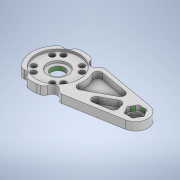
# Autodesk Inventor part: Ankle_side_pitch_frame
Saved by Autodesk Inventor 2020 (Build 240168000, 168)
## iProperties
Part Number: Ankle_side_pitch_frame
Material: アルミニウム 2014-T4
Document SubType Name: Modeling
Designer: Masato Kubotera
Density: 2.8 g/cm^3
Appearance: 滑らか - 淡い灰色
Description: A2017 T4
Mass: 7.07443 g
Surface Area: 29.7848 cm^2
Volume: 2.52658 cm^3
Author: Masato Kubotera
Autodesk Inventor part; units mm, degrees
ref_plane "YZ Plane" through (0, 0, 0) normal (1, 0, 0) x (0, 1, 0)
ref_plane "XZ Plane" through (0, 0, 0) normal (0, 1, 0) x (-1, 0, 0)
ref_plane "XY Plane" through (0, 0, 0) normal (0, 0, 1) x (1, 0, 0)
sketch "スケッチ1" plane through (0, 0, 0) normal (0, 0, 1) x (1, 0, 0)
  circle A0 centre (0, 0) radius 10.5 construction
  circle A1 centre (0, 0) radius 5 construction
  circle A2 centre (0, 0) radius 5.01
  circle A3 centre (0, 0) radius 10.51
  arc A4 (2.1531, 12.3132) -> (2.1531, -12.3132) centre (0, 0) ccw
  circle A5 centre (37.7359, 0) radius 2.75
  arc A6 (38.7694, -5.9103) -> (38.7694, 5.9103) centre (37.7359, 0) ccw
  line L0 (2.1531, 12.3132) -> (38.7694, 5.9103)
  line L1 (2.1531, -12.3132) -> (38.7694, -5.9103)
  line L2 (13.3804, 8.3196) -> (26.7879, 5.9751)
  line L3 (30.7947, -5.2745) -> (23.5904, -6.5342)
  arc A7 (2.1531, -12.3132) -> (-4.7001, 11.5827) centre (0, 0) ccw construction
  arc A8 (38.7694, 5.9103) -> (32.2717, -2.4783) centre (37.7359, 0) ccw construction
  line L4 (34.0196, 4.7105) -> (8.4896, -9.1748) construction
  line L5 (27.399, 2.248) -> (15.2168, -4.3777)
  line L6 (28.8431, 0.7568) -> (22.2903, -2.8072)
  line L7 (32.4358, 4.9875) -> (34.0196, 4.7105) construction
  line L8 (11.5743, -8.6354) -> (8.4896, -9.1748) construction
  arc A9 (31.783, -0.7501) -> (32.2717, -2.4783) centre (37.7359, 0) ccw
  arc A10 (12.2941, -2.2592) -> (11.2378, 5.4737) centre (0, 0) ccw
  line L9 (41.7889, 0) -> (41.2639, -0.9093) construction
  line L10 (39.7624, -3.51) -> (38.7124, -3.51) construction
  line L11 (35.7094, -3.51) -> (35.1844, -2.6007) construction
  line L12 (33.6829, 0) -> (34.2079, 0.9093) construction
  line L13 (35.7094, 3.51) -> (36.7594, 3.51) construction
  line L14 (39.7624, 3.51) -> (40.2874, 2.6007)
  arc A11 (41.2639, -0.9093) -> (41.2639, 0.9093) centre (40.7389, 0) ccw
  arc A12 (40.2874, 2.6007) -> (38.7124, 3.51) centre (39.2374, 2.6007) ccw
  arc A13 (36.7594, 3.51) -> (35.1844, 2.6007) centre (36.2344, 2.6007) ccw
  arc A14 (34.2079, 0.9093) -> (34.2079, -0.9093) centre (34.7329, 0) ccw
  arc A15 (35.1844, -2.6007) -> (36.7594, -3.51) centre (36.2344, -2.6007) ccw
  arc A16 (38.7124, -3.51) -> (40.2874, -2.6007) centre (39.2374, -2.6007) ccw
  line L15 (41.2639, -0.9093) -> (40.2874, -2.6007)
  line L16 (40.2874, -2.6007) -> (39.7624, -3.51) construction
  line L17 (38.7124, -3.51) -> (36.7594, -3.51)
  line L18 (36.7594, -3.51) -> (35.7094, -3.51) construction
  line L19 (35.1844, -2.6007) -> (34.2079, -0.9093)
  line L20 (34.2079, -0.9093) -> (33.6829, 0) construction
  line L21 (35.1844, 2.6007) -> (35.7094, 3.51) construction
  line L22 (34.2079, 0.9093) -> (35.1844, 2.6007)
  line L23 (36.7594, 3.51) -> (38.7124, 3.51)
  line L24 (38.7124, 3.51) -> (39.7624, 3.51) construction
  line L25 (40.2874, 2.6007) -> (41.2639, 0.9093)
  line L26 (41.2639, 0.9093) -> (41.7889, 0) construction
  circle A17 centre (37.7359, 0) radius 2.1
  circle A18 centre (0, 0) radius 3.275
  line L27 (0, 0) -> (27.1359, -16.96) construction
  line L28 (37.7359, 0) -> (27.1359, -16.96) construction
  line L29 (0, 0) -> (37.7359, 0) construction
  line L30 (0, 0) -> (0.848, -0.53)
  line L31 (8.003, 10.918) -> (-6.307, -11.978) construction
  arc A19 (-3.608, -11.968) -> (-7.826, -9.747) centre (-6.307, -11.978) ccw
  arc A20 (5.4321, 11.7398) -> (10.7002, 10.8186) centre (8.003, 10.918) ccw
  arc A21 (13.3804, 8.3196) -> (11.2378, 5.4737) centre (13.0359, 6.3495) ccw
  arc A22 (12.2941, -2.2592) -> (15.2168, -4.3777) centre (14.2612, -2.6207) ccw
  arc A23 (22.2903, -2.8072) -> (23.5904, -6.5342) centre (23.2459, -4.5641) ccw
  arc A24 (30.7947, -5.2745) -> (32.2717, -2.4783) centre (30.4502, -3.3043) ccw
  arc A25 (31.783, -0.7501) -> (28.8431, 0.7568) centre (29.7987, -1.0002) ccw
  arc A26 (27.399, 2.248) -> (26.7879, 5.9751) centre (26.4434, 4.005) ccw
  line L32 (8.003, -10.918) -> (-6.307, 11.978) construction
  arc A27 (-7.826, 9.747) -> (-3.608, 11.968) centre (-6.307, 11.978) ccw
  arc A28 (10.7002, -10.8186) -> (5.4321, -11.7398) centre (8.003, -10.918) ccw
  line L33 (-6.625, -10.6) -> (6.625, 10.6) construction
  circle A29 centre (4.505, 7.208) radius 1.35
  circle A30 centre (-7.208, 4.505) radius 1.35
  circle A31 centre (-4.505, -7.208) radius 1.35
  circle A32 centre (7.208, -4.505) radius 1.35
  circle A33 centre (4.505, -7.208) radius 1.35
  circle A34 centre (-7.208, -4.505) radius 1.35
  circle A35 centre (-4.505, 7.208) radius 1.35
  circle A36 centre (7.208, 4.505) radius 1.35
  circle A37 centre (-4.505, -7.208) radius 2.4 construction
  point P0 (8.4896, 9.1748)
  point P1 (34.0196, -4.7105)
  point P2 (10.3333, -7.0337)
  point P3 (32.3635, 2.6714)
  point P4 (39.7624, 3.51)
  point P5 (9.5861, 8.9831)
  point P6 (9.0332, 8.6401)
  point P7 (-3.608, 11.968)
  dimension "d0" = 21
  dimension "d1" = 10
  dimension "d2" = 0.01
  dimension "d3" = 0.01
  dimension "d4" = 25
  dimension "d7" = 5.5
  dimension "d8" = 6
  dimension "d15" = 2
  dimension "d16" = 2
  dimension "d17" = 1
  dimension "d18" = 1
  dimension "d20" = 1.05
  dimension "d23" = 360
  dimension "d25" = 7.02
  dimension "d30" = 4.2
  dimension "d33" = 6.55
  dimension "d41" = 20
  dimension "d42" = 32
  dimension "d46" = 27
  dimension "d47" = 1
  dimension "d48" = 90
  dimension "d49" = 2.699
  dimension "d50" = 2.699
  dimension "d51" = 2
  dimension "d52" = 2
  dimension "d53" = 2
  dimension "d55" = 2.699
  dimension "d56" = 2.699
  dimension "d57" = 2.7
  dimension "d58" = 8.5
  dimension "d61" = 360
  dimension "d63" = 4.8
  constraints: 68 end point, 62 point on circle, 38 centre point, 20 coincident, 17 tangent, 14 point on line, 7 parallel, 6 symmetric about line, 3 collinear, 3 equal radius, 2 midpoint, 2 perpendicular, 1 horizontal, 57 other
  measures "d0" diameter of A0
  measures "d1" diameter of A1
  measures "d2" radial gap between concentric circles of A3 A0
  measures "d3" radial gap between concentric circles of A2 A1
  measures "d4" diameter of A4
  measures "d7" diameter of A5
  measures "d8" radius of A6
  measures "d15" distance between parallel lines of L0 L2
  measures "d16" distance between parallel lines of L1 L3
  measures "d17" distance between parallel lines of L4 L6
  measures "d18" distance between parallel lines of L5 L4
  measures "d20" radius of A11
  measures "d25" distance between parallel lines of L23 L17
  measures "d30" diameter of A17
  measures "d33" diameter of A18
  measures "d41" distance of L28.start L27.end
  measures "d42" distance of L27.start L27.end
  measures "d46" distance of L31.start L31.end
  measures "d47" distance of L30.start L30.end
  measures "d48" angle of L27 L31
  measures "d49" radius of A19
  measures "d50" radius of A20
  measures "d51" radius of A21
  measures "d52" radius of A24
  measures "d53" radius of A26
  measures "d55" radius of A27
  measures "d56" radius of A28
  measures "d57" diameter of A29
  measures "d58" distance of point (0, 0) A29.centre
  measures "d63" diameter of A37
extrude "押し出し1" add sketch "スケッチ1" along normal blind 4 contours L0 A20 A6 L1 A28 A4 A19 A27
extrude "押し出し2" add sketch "スケッチ1" along normal blind 1.6 contours A12 L14 | L14 L25 A11 L15 A16 L17 A15 L19 A14 L22 A13 L23 A12
extrude "押し出し3" add sketch "スケッチ1" along normal blind 1 contours A5
extrude "押し出し4" add sketch "スケッチ1" along normal blind 3 contours A3
extrude "押し出し5" add sketch "スケッチ1" along normal blind 2 contours A2
extrude "押し出し6" add sketch "スケッチ1" along normal blind 1 contours L2 A26 L5 A22 A10 A21 | L3 A23 L6 A25 A9 A24
fillet "フィレット1" radius 2 8 edges at (-3.608, -11.968, 2) (-7.826, -9.747, 2) (10.7002, 10.8186, 2) (5.4321, 11.7398, 2) (5.4321, -11.7398, 2) (10.7002, -10.8186, 2) (-7.826, 9.747, 2) (-3.608, 11.968, 2)
equation "\"d3\" = d2"
equation "\"d18\" = d17"
equation "\"d50\" = d49"
